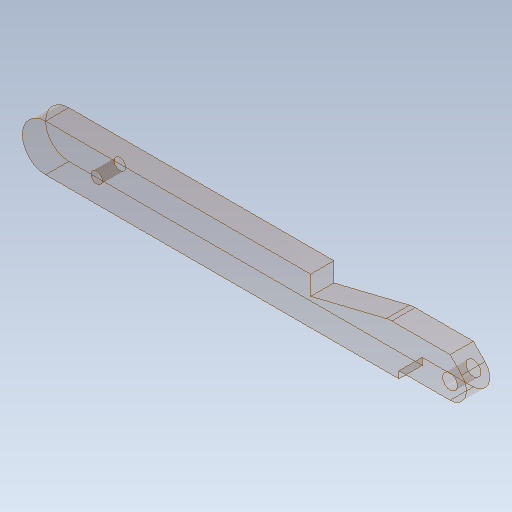
# Autodesk Inventor part: カウンター
Saved by Autodesk Inventor 2020.2 (Build 242310000, 310)
## iProperties
Created: 2020-04-03
Part Number: カウンター
Material: ポリカーボネート、スモーク
Document SubType Name: Modeling
Designer: aoyama
Density: 1.2 g/cm^3
Appearance: ポリカーボネート - スモーク
Mass: 5.19336 g
Surface Area: 28.5877 cm^2
Volume: 4.3278 cm^3
Author: aoyama
Autodesk Inventor part; units mm, degrees
ref_plane "YZ Plane" through (0, 0, 0) normal (1, 0, 0) x (0, 1, 0)
ref_plane "XZ Plane" through (0, 0, 0) normal (0, 1, 0) x (-1, 0, 0)
ref_plane "XY Plane" through (0, 0, 0) normal (0, 0, 1) x (1, 0, 0)
sketch "スケッチ1" plane through (0, 0, 0) normal (0, 0, 1) x (1, 0, 0)
  line L0 (0, 0) -> (-92, 0) construction
  line L1 (0, 5) -> (-92, 5)
  line L2 (-92, -5) -> (0, -5)
  arc A0 (0, -5) -> (0, 5) centre (0, 0) ccw
  circle A1 centre (0, 0) radius 1.6
  line L3 (-29.5, 1.5) -> (-29.5, 6.5)
  line L4 (-29.5, 1.5) -> (17.5, 13.0396)
  line L5 (17.5, 13.0396) -> (17.5, 18.1985)
  line L6 (17.5, 18.1985) -> (-29.5, 6.5)
  circle A2 centre (0, 15) radius 1.5
  line L7 (0, 15) -> (0, 0)
  circle A3 centre (0, 15) radius 2.5
  circle A4 centre (15, 15) radius 2.5
  circle A5 centre (15, 15) radius 1.5
  line L8 (-30, 6.8908) -> (-30, 0.8624)
  line L9 (-30, 0.8624) -> (18, 12.6475)
  line L10 (18, 12.6475) -> (18, 18.8382)
  line L11 (18, 18.8382) -> (-30, 6.8908)
  line L12 (-92, 5) -> (-92, -5)
  line L13 (0, 0) -> (-11, 0)
  line L14 (-11, 0) -> (-11, -3.5)
  line L15 (-11, 0) -> (-7.5, 0) construction
  line L16 (-11, -3.5) -> (0, -3.5)
  circle A6 centre (0, 0) radius 3.5
  line L17 (0, 5) -> (2.4995, 2.45)
  line L18 (-11, 0) -> (-11, -5)
  line L19 (15, 15) -> (15, 15)
  circle A7 centre (15, 15) radius 1.5
  circle A8 centre (15, 15) radius 2.5
  line L20 (-67.5, 5) -> (-67.5, -5)
  point P0 (-15.2447, 5)
  point P1 (-29.5, 5)
  point P2 (0, 12.5)
  point P3 (0.6029, 12.5738)
  point P4 (0, 8.7429)
  point P5 (2.4387, 14.4497)
  point P6 (-1.8962, 13.3707)
  point P7 (-13.1477, 5)
  point P8 (-30, 5)
  point P9 (-11, -4.9654)
  dimension "d14" = 10
  dimension "d1" = 92
  dimension "d2" = 3.2
  dimension "d3" = 5
  dimension "d4" = 3
  dimension "d5" = 15
  dimension "d6" = 1
  dimension "d11" = 15
  dimension "d16" = 0.5
  dimension "d24" = 5
  dimension "d25" = 11
  dimension "d26" = 90
  dimension "d27" = 7
  dimension "d30" = 0
  dimension "d31" = 3
  dimension "d32" = 1
  dimension "d33" = 62
  dimension "d34" = 37.5
  dimension "d46" = 92
  dimension "d47" = 3.5
  constraints: 44 end point, 9 centre point, 7 tangent, 6 vertical, 5 horizontal, 5 point on line, 4 point on circle, 3 coincident, 1 parallel, 1 perpendicular, 6 other
  measures "d1" distance of L0.end L0.start
  measures "d2" diameter of A1
  measures "d3" distance of L3.start L3.end
  measures "d4" diameter of A2
  measures "d5" distance of L7.start L7.end
  measures "d6" radial gap between concentric circles of A2 A3
  measures "d11" distance of L7.start L19.start
  measures "d16" distance between parallel lines of L3 L8
  measures "d24" radius of A0
  measures "d25" distance of L13.end L7.end
  measures "d26" angle of L14 L15
  measures "d27" diameter of A6
  measures "d30" distance of L19.start L19.end
  measures "d31" diameter of A7
  measures "d32" radial gap between concentric circles of A7 A8
  measures "d33" distance from line of L1.end L8
  measures "d34" distance between parallel lines of L8 L20
  measures "d46" distance between parallel lines of L7 L12
  measures "d47" distance from line of L1 L3.start
extrude "押し出し1" add sketch "スケッチ1" along normal blind 5 contours L20 L2 L12 L1 | L1 L8 L9 L7 A6 L13 L14 L18 L2 L20 | L14 L13 A6 L16 | L17 A6 L7 | A6 L13 A1 L7 | L7 A1 L13 A6
fillet "フィレット1" radius 5 2 edges at (-92, 5, 2.5) (-92, -5, 2.5)
fillet "フィレット2" radius 5 1 edges at (-13.1477, 5, 2.5)
sketch "スケッチ3" plane through (0, 0, 5) normal (0, 0, 1) x (1, 0, 0)
  arc A0 (-12.5429, 5) -> (-13.7351, 4.8558) centre (-12.5429, 0) ccw projected
  line L0 (-13.7351, 4.8558) -> (-30, 0.8624) projected
  line L1 (-30, 0.8624) -> (-30, 5) projected
  line L2 (-30, 5) -> (-87, 5) projected
  arc A1 (-87, 5) -> (-87, -5) centre (-87, 0) ccw projected
  line L3 (-87, -5) -> (-11, -5) projected
  line L4 (-11, -5) -> (-11, -3.5) projected
  line L5 (-11, -3.5) -> (0, -3.5) projected
  arc A2 (0, -3.5) -> (2.4995, 2.45) centre (0, 0) ccw projected
  line L6 (2.4995, 2.45) -> (0, 5) projected
  line L7 (0, 5) -> (-12.5429, 5) projected
  circle A3 centre (0, 0) radius 1.6 projected
  circle A4 centre (-76, 0) radius 1.25
  dimension "d49" = 2.5
  dimension "d50" = 11
  constraints: 1 centre point
  measures "d49" diameter of A4
  measures "d50" distance of A4.centre A1.centre
extrude "押し出し3" cut sketch "スケッチ3" against normal blind 10 contours A4
thread "ねじ3" size "M3x0.5" class "6H" standard "ANSI Metric M Profile" full length
